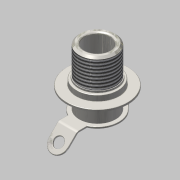
# Autodesk Inventor part: InputJack_shield
Saved by Autodesk Inventor 2015 SP1 (Build 190203100, 203)
## iProperties
Created: 2015-06-13
Part Number: InputJack_shield
Material: Generic
Document SubType Name: Modeling
Designer: Peter Mulkers
Density: 1 g/cm^3
Appearance: Titanium
Sheet Metal Rule: Default
Author: Peter Mulkers
Autodesk Inventor part; units mm, degrees
ref_plane "YZ Plane" through (0, 0, 0) normal (1, 0, 0) x (0, 1, 0)
ref_plane "XZ Plane" through (0, 0, 0) normal (0, 1, 0) x (-1, 0, 0)
ref_plane "XY Plane" through (0, 0, 0) normal (0, 0, 1) x (1, 0, 0)
sketch "Sketch1" plane through (0, 0, 0) normal (0, 0, 1) x (1, 0, 0)
  circle A0 centre (0, 0) radius 4.7625
  dimension "d0" = 9.525
  constraints: 1 centre point, 1 coincident
  measures "d0" diameter of A0
extrude "Extrusion1" add sketch "Sketch1" along normal blind 7.5
sketch "Sketch2" plane through (0, 0, 7.5) normal (0, 0, 1) x (1, 0, 0)
  circle A0 centre (0, 0) radius 4.9
  dimension "d3" = 9.8
  constraints: 1 centre point, 1 coincident
  measures "d3" diameter of A0
extrude "Extrusion2" add sketch "Sketch2" along normal blind 0.5
sketch "Sketch3" plane through (0, 0, 8) normal (0, 0, 1) x (1, 0, 0)
  circle A0 centre (0, 0) radius 5.5
  dimension "d6" = 11
  constraints: 1 centre point, 1 coincident
  measures "d6" diameter of A0
extrude "Extrusion3" add sketch "Sketch3" along normal blind 1.5
sketch "Sketch4" plane through (0, 0, 9.5) normal (0, 0, 1) x (1, 0, 0)
  circle A0 centre (0, 0) radius 8
  dimension "d9" = 16
  constraints: 1 centre point, 1 coincident
  measures "d9" diameter of A0
extrude "Extrusion4" add sketch "Sketch4" along normal blind 0.5
sketch "Sketch5" plane through (0, 0, 10) normal (0, 0, 1) x (1, 0, 0)
  circle A0 centre (0, 0) radius 4.7625
  dimension "d12" = 9.525
  constraints: 1 centre point, 1 coincident
  measures "d12" diameter of A0
extrude "Extrusion5" add sketch "Sketch5" along normal blind 5
sketch "Sketch6" plane through (0, 0, 15) normal (0, 0, 1) x (1, 0, 0)
  line L0 (1.25, -7.5) -> (-1.25, -7.5)
  line L1 (2.5, 7.5) -> (-2.5, 7.5)
  line L2 (2.5, 7.5) -> (2.5, 5.1781)
  line L3 (-2.5, 7.5) -> (-2.5, 5.1781)
  line L4 (1.25, -7.5) -> (1.25, -7)
  line L5 (-1.25, -7.5) -> (-1.25, -7)
  line L6 (1.25, -7) -> (4.1475, -3.9826)
  line L7 (-1.25, -7) -> (-4.1475, -3.9826)
  arc A0 (4.1475, -3.9826) -> (2.5, 5.1781) centre (0, 0) ccw
  arc A1 (-2.5, 5.1781) -> (-4.1475, -3.9826) centre (0, 0) ccw
  point P0 (0, -7.5)
  point P1 (0, 7.5)
  dimension "d35" = 2.5
  dimension "d36" = 7.5
  dimension "d37" = 5
  dimension "d38" = 7.5
  dimension "d52" = 0.5
  dimension "d53" = 0.5
  dimension "d54" = 5.75
  dimension "d55" = 5.75
  constraints: 16 end point, 4 point on circle, 4 vertical, 2 centre point, 2 horizontal, 2 midpoint, 2 tangent, 2 vertical alignment, 1 coincident
  measures "d35" distance of L0.start L0.end
  measures "d36" distance from line of point (0, 0) L0
  measures "d37" distance of L1.start L1.end
  measures "d38" distance from line of point (0, 0) L1
  measures "d52" distance of L0.start L4.end
  measures "d53" distance of L0.end L5.end
  measures "d54" radius of A0
  measures "d55" radius of A1
extrude "Extrusion6" add sketch "Sketch6" along normal blind 0.5
sketch "Sketch7" plane through (0, 0, 0) normal (0, 0, -1) x (-1, 0, 0)
  circle A0 centre (0, 0) radius 3.25
  dimension "d18" = 6.5
  constraints: 1 centre point, 1 coincident
  measures "d18" diameter of A0
extrude "Extrusion7" cut sketch "Sketch7" against normal up to surface (15.5 mm away)
sketch "Sketch8" plane through (0, 0, 15.5) normal (0, 0, 1) x (-0.2126674, 0.9771246, 0)
  circle A0 centre (0, 0) radius 4.25
  circle A1 centre (0, 0) radius 3.25
  dimension "d56" = 8.5
  dimension "d57" = 6.5
  constraints: 2 centre point, 2 coincident
  measures "d56" diameter of A0
  measures "d57" diameter of A1
extrude "Extrusion8" add sketch "Sketch8" along normal blind 0.5
fillet "Fillet1" radius 0.5 2 edges at (0.6912, -3.1757, 16) (0.9038, -4.1528, 16)
thread "Thread1" size "3/8-32 UNEF" class "2A" standard "ANSI Unified Screw Threads" full length
chamfer "Chamfer1" distance 0.5 angle 45 1 edges at (-4.7625, 0, 0)
fillet "Fillet2" radius 0.5 1 edges at (3.25, 0, 0)
fillet "Fillet3" radius 0.15 4 edges at (-5.5, 0, 8) (-5.5, 0, 9.5) (-8, 0, 9.5) (-4.9, 0, 8)
sketch "Sketch10" plane through (2.5, 7.5, 15.5) normal (0, 0.7071068, -0.7071068) x (-1, 0, 0)
  line L0 (5, 0) -> (0, 0)
  line L1 (0, 0) -> (0, -5.7929)
  line L2 (0, -5.7929) -> (5, -5.7929)
  line L3 (5, -5.7929) -> (5, 0)
  constraints: 6 end point, 1 horizontal, 1 perpendicular, 1 vertical
edge flange "Flange1" height 6 angle -45 thickness 0.5 bend radius 0.5 thickness toward (0, 0.7071068, -0.7071068) relief tear relief width 0.5 relief depth 0.25 edges at (0, 7.5, 15) wall of the first edge with corners at (-2.5, 7.5, 15.5) (2.5, 7.5, 15.5) (2.5, 11.5962, 19.5962) (-2.5, 11.5962, 19.5962)
bend "Bend1"
corner "Corner1"
fillet "Corner Round1" radius 2.5 2 edges at (-2.5, 11.773, 19.4194) (2.5, 11.773, 19.4194)
sketch "Sketch11" plane through (-1.25, -7.5, 15) normal (0, -1, 0) x (1, 0, 0)
  line L0 (2.5, 0) -> (0, 0)
  line L1 (0, 0) -> (0, -0.75)
  line L2 (0, -0.75) -> (2.5, -0.75)
  line L3 (2.5, -0.75) -> (2.5, 0)
  constraints: 6 end point, 1 horizontal, 1 perpendicular, 1 vertical
edge flange "Flange2" height 1.25 angle 90 thickness 0.5 bend radius 0.5 thickness toward (0, -1, 0) relief tear relief width 0.5 relief depth 0.25 edges at (0, -7.5, 15) wall of the first edge with corners at (1.25, -7.5, 15) (-1.25, -7.5, 15) (-1.25, -7.5, 14.25) (1.25, -7.5, 14.25)
bend "Bend2"
corner "Corner2"
fillet "Fillet4" radius 0.15 30 edges at (-2.6987, -5.4913, 15.5) (-5.6592, 1.0178, 15.5) (5.6592, 1.0178, 15.5) (2.6987, -5.4913, 15.5) (2.5, 7.4842, 15.5381) (2.5, 8.7375, 16.7375) (-1.7678, 11.0784, 19.0784) (-2.5, 8.7375, 16.7375) (-2.5, 7.4842, 15.5381) (-2.5, 6.2355, 15.5) (2.5, 6.2355, 15.5) (-1.7678, 11.432, 18.7249) (2.5, 9.091, 16.3839) (2.5, 7.6756, 15.0761) (2.5, 6.2355, 15) (-2.5, 7.6756, 15.0761) (-2.5, 6.2355, 15) (-2.5, 9.091, 16.3839) (-2.6987, -5.4913, 15) (-5.6592, 1.0178, 15) (5.6592, 1.0178, 15) (2.6987, -5.4913, 15) (-1.25, -8, 14.375) (-1.25, -7.7071, 15.2071) (-1.25, -7.5, 14.375) (-1.25, -7.3536, 14.8536) (1.25, -8, 14.375) (1.25, -7.7071, 15.2071) (1.25, -7.5, 14.375) (1.25, -7.3536, 14.8536)
sketch "Sketch12" plane through (0, 9.8284, 17.8284) normal (0, -0.7071068, 0.7071068) x (1, 0, 0)
  line L0 (-2.35, -3.0858) -> (-2.35, 0) projected
  line L1 (-2.35, -3.0858) -> (2.35, -3.0858) projected
  line L2 (2.35, 0) -> (2.35, -3.0858) projected
  arc A0 (2.35, 0) -> (-2.35, 0) centre (0, 0) ccw projected
  circle A1 centre (0, 0) radius 1.25
  point P0 (0, -19.5563)
  dimension "d69" = 2.5
  constraints: 1 centre point, 1 coincident
  measures "d69" diameter of A1
extrude "Extrusion9" cut sketch "Sketch12" against normal blind 0.5 contours A1
fillet "Fillet5" radius 0.15 2 edges at (-1.25, 9.8284, 17.8284) (-1.25, 10.182, 17.4749)
equation "\"d41\" = BendReliefWidth"
equation "\"d42\" = BendReliefDepth"
equation "\"d43\" = MinimumRemnant"
equation "\"d44\" = BendRadius"
equation "\"d47\" = BendRadius"
equation "\"d48\" = CornerReliefSize"
equation "\"d49\" = GapSize"
equation "\"d50\" = JacobiRadiusSize"
equation "\"d58\" = BendReliefWidth"
equation "\"d59\" = BendReliefDepth"
equation "\"d60\" = MinimumRemnant"
equation "\"d61\" = BendRadius"
equation "\"d64\" = BendRadius"
equation "\"d65\" = CornerReliefSize"
equation "\"d66\" = GapSize"
equation "\"d67\" = JacobiRadiusSize"
equation "\"BendRadius\" = Thickness"
equation "\"BendReliefWidth\" = Thickness"
equation "\"BendReliefDepth\" = 0.5 * Thickness"
equation "\"CornerReliefSize\" = 4 * Thickness"
equation "\"MinimumRemnant\" = 2 * Thickness"
equation "\"TransitionRadius\" = BendRadius"
equation "\"JacobiRadiusSize\" = BendRadius"
equation "\"GapSize\" = Thickness"
equation "\"Thickness\" = 0.5"
body "Solid1"
